Autodesk Fusion 360 part; units mm, degrees
note: some values were not read from the file. Chosen so that the rebuilt part matches the saved one: which pieces of a blend or face edit are solid.
(part 5 of 5)
equation "d614 = button_screwd"
equation "d616 = lcd_boardh / 2"
equation "d617 = poti_screwd"
equation "d619 = lcd_boardh / 2"
equation "d620 = lcd_screwd / 2 + lcd_blockdistx"
equation "d621 = lcd_screwd / 2 + lcd_blockdistx"
equation "d622 = lcd_screwd / 2 + lcd_blockdisty"
equation "d623 = lcd_screwd / 2 + lcd_blockdisty"
equation "d626 = top3_bezel"
equation "d627 = top3_bezel"
equation "d633 = box_iw - 2 * ( top3_bezel + screwd )"
equation "d634 = -( box_ih - 2 * ( top3_bezel + screwd ) )"
equation "brk_btn_switchd = 2 mm"
equation "btk_btn_udbdist_short = 3 mm"
equation "brk_aux_jacknubdist = 4 mm"
equation "d664 = aux_d"
equation "d665 = aux_dist"
equation "d667 = brk_aux_jacknubdist"
equation "aux_sd_topplatedist = 6 mm"
equation "d669 = aux_sd_topplatedist"
equation "pcbthickness = 1 mm"
equation "d671 = aux_d / 2 + pcbthickness"
equation "d672 = sdcard_thickness"
equation "d673 = sdcard_w"
equation "sdcard_thickness = 2 mm"
equation "sdcard_w = 24 mm"
equation "d677 = wallthickness + top3_bezel + 2 * screwd"
equation "d678 = top3_bezel + 2 * screwd"
equation "d679 = wallthickness + top3_bezel"
equation "d680 = top3_bezel + 2 * screwd"
equation "d681 = top3_bezel + 2 * screwd"
equation "d684 = top3_bezel + 2 * screwd"
equation "d689 = -box_id"
equation "odd_frontoverhang = 21 mm"
equation "d692 = odd_w"
equation "d693 = odd_frontoverhang"
equation "d699 = odd_d"
equation "d702 = odd_inset_w"
equation "d703 = odd_inset_d"
equation "d704 = odd_w"
equation "d705 = odd_w"
equation "d706 = odd_frontoverhang"
equation "d707 = odd_d"
equation "d710 = odd_w"
equation "d711 = odd_d"
equation "d712 = odd_inset_w"
equation "d713 = odd_inset_d"
equation "d714 = odd_w"
equation "d715 = odd_inset_w"
equation "d716 = odd_inset_d"
equation "d718 = wallthickness"
equation "d719 = odd_w * 0.75"
equation "d742 = wallthickness"
equation "d743 = wallthickness"
equation "d788 = -( box_ih - cornerdim )"
equation "d789 = -( box_id - cornerdim )"
equation "d791 = top3_bezel"
equation "d792 = 2 * top3_bezel"
equation "d793 = 2 * top3_bezel"
equation "d796 = box_ih - cornerdim"
equation "d797 = box_id - cornerdim"
equation "d808 = box_id"
equation "ledstrip_w = 11 mm"
equation "ledstrip_thickness = 3 mm"
equation "d816 = box_id"
equation "d817 = box_iw"
equation "d818 = box_iw - 4 * ledstrip_thickness"
equation "d820 = 2 * ledstrip_thickness"
equation "d821 = 2 * ledstrip_thickness"
equation "d822 = box_iw - 2 * ledstrip_thickness"
equation "d823 = box_id - 2 * ledstrip_thickness"
equation "d826 = wallthickness"
equation "d840 = wallthickness"
equation "d841 = wallthickness"
equation "d843 = odd_h"
equation "d848 = wallthickness"
equation "d854 = ledstrip_w"
equation "d856 = wallthickness"
equation "d859 = box_iw"
equation "d862 = wallthickness"
equation "d865 = box_iw"
equation "d867 = ledstrip_w"
equation "d868 = box_iw"
equation "sidepiece_oddled_l = platethickness + ledstrip_w + 3 * wallthickness"
equation "d884 = wallthickness + platethickness"
equation "d885 = odd_h"
equation "d887 = wallthickness"
equation "d890 = wallthickness"
equation "d894 = -box_id"
equation "d898 = top3_bezel"
equation "d899 = platethickness"
equation "d904 = ( wallthickness - plasticthickness ) / 2"
equation "d920 = -box_ih"
equation "d921 = wallthickness"
equation "d922 = ( wallthickness - platethickness ) / 2"
equation "d923 = platethickness"
equation "d929 = longnotchleadin"
equation "d930 = wallthickness"
equation "d931 = longnotchleadin"
equation "d932 = wallthickness"
equation "d933 = longnotchleadin"
equation "d934 = wallthickness"
equation "d937 = wallthickness"
equation "d938 = box_ih / 2"
equation "d939 = ledstrip_thickness"
equation "d940 = ledstrip_thickness"
equation "d948 = wallthickness"
equation "d949 = wallthickness"
equation "d951 = wallthickness"
equation "d954 = box_iw"
equation "d956 = longnotchleadin"
equation "d971 = cornerdim"
equation "d972 = cornerdim"
equation "d973 = cornerdim + wallthickness + plasticthickness + platethickness"
equation "d974 = cornerdim + wallthickness + plasticthickness + platethickness"
equation "d975 = cornerdim + wallthickness"
equation "d976 = cornerdim + wallthickness"
equation "d977 = platethickness"
equation "d980 = platethickness"
equation "d981 = ( wallthickness - platethickness ) / 2"
equation "d982 = platethickness"
equation "d987 = plasticthickness"
equation "d989 = plasticthickness + platethickness + wallthickness + cornerdim"
equation "d991 = platethickness + plasticthickness + wallthickness + top3_bezel"
equation "d993 = screwd"
equation "d994 = screwd"
equation "d995 = cornerdim / 2"
equation "d996 = cornerdim / 2"
equation "d997 = cornerdim / 2"
equation "d998 = cornerdim / 2"
equation "d999 = screwd"
equation "d1000 = screwd"
equation "d1001 = cornerdim / 2"
equation "d1002 = cornerdim / 2"
equation "d1003 = cornerdim / 2"
equation "d1004 = cornerdim / 2"
equation "d1009 = cornerdim + wallthickness + plasticthickness"
equation "d1010 = 2 * cornerdim + platethickness + wallthickness"
equation "d1011 = cornerdim + wallthickness"
equation "d1012 = screwd"
equation "d1013 = cornerdim / 2"
equation "d1014 = cornerdim / 2"
equation "d1015 = screwd"
equation "d1016 = cornerdim / 2"
equation "d1017 = cornerdim / 2"
equation "d1018 = screwd"
equation "d1019 = screwd"
equation "d1020 = cornerdim / 2"
equation "d1021 = cornerdim / 2"
equation "d1022 = cornerdim / 2"
equation "d1023 = cornerdim / 2"
equation "d1024 = screwd"
equation "d1025 = screwd"
equation "d1030 = wallthickness"
named bodies: "corner3o", "corner3i", "corner2o", "corner2i", "3to8_r", "3plate_l", "3plate_r", "3to8_l", "corner2o_long"
